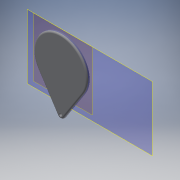
# Autodesk Inventor part: trapdoor_servo
Saved by Autodesk Inventor 2019 (Build 230136000, 136)
## iProperties
Created: 2019-01-09
Part Number: trapdoor_servo
Material: Generic
Document SubType Name: Modeling
Designer: jmc
Density: 1 g/cm^3
Appearance: Default
Author: jmc
Autodesk Inventor part; units mm, degrees
ref_plane "YZ Plane" through (0, 0, 0) normal (1, 0, 0) x (0, 1, 0)
ref_plane "XZ Plane" through (0, 0, 0) normal (0, 1, 0) x (-1, 0, 0)
ref_plane "XY Plane" through (0, 0, 0) normal (0, 0, 1) x (1, 0, 0)
ref_plane "Work Plane1" through (0, 0, 0) normal (0, 0, -1) x (-1, 0, 0)
ref_plane "Work Plane3" through (-59.1654, 22.8024, -1.2767) normal (0, 0, 1) x (0, 1, 0)
sketch "Sketch3" plane through (-59.1654, 22.8024, -1.2767) normal (0, 0, 1) x (0, 1, 0)
  circle A0 centre (0, 0) radius 25.15 construction
  arc A1 (-13.6627, -21.1152) -> (-13.6627, 21.1152) centre (0, 0) ccw construction
  arc A2 (-13.6627, -21.1152) -> (-13.6627, 21.1152) centre (0, 0) ccw
  line L0 (0, 0) -> (-40, 0) construction
  circle A3 centre (-40, 0) radius 1.42 construction
  circle A4 centre (-40, 0) radius 1.42
  arc A5 (-41.8579, 2.8713) -> (-41.8579, -2.8713) centre (-40, 0) ccw
  line L1 (-41.8579, 2.8713) -> (-13.6627, 21.1152)
  line L2 (-41.8579, -2.8713) -> (-13.6627, -21.1152)
  point P0 (-22.8024, -59.1654)
  dimension "d2" = 40
  dimension "d3" = 2.84
  dimension "d4" = 2
  constraints: 6 end point, 6 point on circle, 5 centre point, 5 coincident, 4 tangent, 3 concentric, 1 horizontal
  measures "d2" distance of L0.start L0.end
  measures "d3" diameter of A3
  measures "d4" radial gap between concentric circles of A5 A3
extrude "Extrusion1" add sketch "Sketch3" along normal blind 2.4
fillet "Fillet1" radius 1.6 4 edges at (-71.1587, -4.9579, 1.1233) (-59.1654, -20.6176, 1.1233) (-47.1721, -4.9579, 1.1233) (-59.1654, 47.9524, 1.1233)
body "Solid1"
